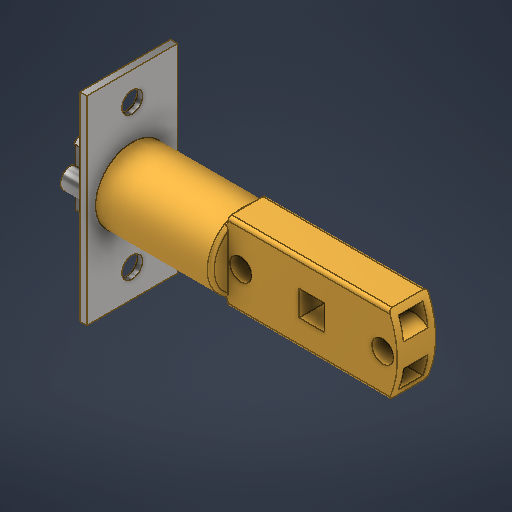
# Autodesk Inventor part: LOK-58 LLAVIN DE POMO (PASADOR)
Saved by Autodesk Inventor 2025 (Build 290162000, 162)
## iProperties
Created: 2026-02-18
Part Number: LOK-58 LLAVIN DE POMO (PASADOR)
Material: Latón, amarillo claro
Document SubType Name: Modeling
Designer: ROLANDO
Density: 8.47 g/cm^3
Appearance: Latón - Satinado
Author: ROLANDO
Autodesk Inventor part; units mm, degrees
ref_plane "YZ Plane" through (0, 0, 0) normal (1, 0, 0) x (0, 1, 0)
ref_plane "XZ Plane" through (0, 0, 0) normal (0, 1, 0) x (-1, 0, 0)
ref_plane "XY Plane" through (0, 0, 0) normal (0, 0, 1) x (1, 0, 0)
sketch "Boceto1" plane through (0, 0, 0) normal (0, 0, 1) x (1, 0, 0)
  circle A0 centre (20.35, 0) radius 3.15
  circle A1 centre (-20.35, 0) radius 3.15
  line L0 (-3.65, 3.65) -> (3.65, 3.65)
  line L1 (3.65, 3.65) -> (3.65, -3.65)
  line L2 (3.65, -3.65) -> (-3.65, -3.65)
  line L3 (-3.65, -3.65) -> (-3.65, 3.65)
  line L4 (-3.65, 3.65) -> (3.65, -3.65) construction
  line L5 (3.65, 3.65) -> (-3.65, -3.65) construction
  line L6 (-24, 11.25) -> (22, 11.25)
  line L7 (22, -11.25) -> (-24, -11.25)
  line L8 (-24, -11.25) -> (-24, 11.25)
  arc A2 (22, -11.25) -> (22, 11.25) centre (-2.0625, 0) ccw
  point P0 (0, 0)
  point P1 (0, 0)
  point P2 (0, 0)
  dimension "d1" = 6.3
  dimension "d2" = 6.3
  dimension "d3" = 7.3
  dimension "d4" = 7.3
  dimension "d7" = 46
  dimension "d8" = 24
  dimension "d9" = 22.5
  dimension "d10" = 11.25
  dimension "d12" = 1
  dimension "d13" = 46
  dimension "d15" = 3.65
  dimension "d16" = 40.7
  dimension "d17" = 20.35
  constraints: 18 end point, 3 centre point, 2 coincident, 2 horizontal, 2 horizontal alignment, 2 midpoint, 2 parallel, 2 perpendicular, 2 point on circle
  measures "d1" diameter of A0
  measures "d2" diameter of A1
  measures "d3" distance of L1.end L2.end
  measures "d4" distance of L0.end L1.end
  measures "d7" distance of L7.start L7.end
  measures "d8" distance from line of point (0, 0) L8
  measures "d9" distance of L7.end L6.start
  measures "d10" distance from line of point (0, 0) L6
  measures "d13" distance of L6.start L6.end
  measures "d15" distance from line of A1.centre L8
  measures "d16" distance of A1.centre A0.centre
  measures "d17" distance of point (0, 0) A0.centre
extrude "Extrusión1" add sketch "Boceto1" against normal blind 11
sketch "Boceto2" plane through (-24, -11.25, 0) normal (-1, 0, 0) x (0, 0, 1)
  circle A0 centre (-5.5, 11.25) radius 10.5
  line L0 (0, 0) -> (-11, 0) projected
  line L1 (0, 22.5) -> (0, 0) projected
  point P0 (0, 11.25)
  dimension "d20" = 21
  dimension "d21" = 11.25
  dimension "d22" = 5.5
  constraints: 1 centre point
  measures "d20" diameter of A0
  measures "d21" distance from line of L0 A0.centre
  measures "d22" distance from line of L1 A0.centre
extrude "Extrusión2" add sketch "Boceto2" along normal blind 33
sketch "Boceto3" plane through (-57, 0, -5.5) normal (-1, 0, 0) x (0, 0, 1)
  line L0 (-13, 28.5) -> (13, 28.5)
  line L1 (13, 28.5) -> (13, -28.5)
  line L2 (13, -28.5) -> (-13, -28.5)
  line L3 (-13, -28.5) -> (-13, 28.5)
  line L4 (-13, 28.5) -> (13, -28.5) construction
  line L5 (13, 28.5) -> (-13, -28.5) construction
  circle A0 centre (0, 0) radius 10.5 projected
  line L6 (6.5, -8.2462) -> (6.5, -3.1943)
  line L7 (6.5, 8.2462) -> (6.5, 3.1943)
  line L8 (10.2924, 0) -> (-1.6343, 0) construction
  arc A1 (6.5, -3.1943) -> (6.5, 3.1943) centre (7, 0) ccw
  arc A2 (6.5, -8.2462) -> (6.5, 8.2462) centre (0, 0) ccw construction
  point P0 (5.5, 0)
  dimension "d25" = 26
  dimension "d26" = 57
  dimension "d27" = 13
  dimension "d29" = 28.5
  dimension "d68" = 6.5
  dimension "d69" = 3.2332
  dimension "d72" = 0.5
  constraints: 18 end point, 4 point on circle, 2 centre point, 2 horizontal, 2 midpoint, 2 parallel, 1 collinear, 1 perpendicular, 1 point on line, 1 vertical
  measures "d25" distance of L1.end L2.end
  measures "d26" distance of L0.end L1.end
  measures "d27" distance from line of A0.centre L1
  measures "d29" distance from line of L0 A0.centre
  measures "d68" distance from line of point (0, 0) L6
  measures "d69" radius of A1
  measures "d72" distance from line of L6 A1.centre
extrude "Extrusión3" add sketch "Boceto3" along normal blind 2 contours L0 L1 L2 L3 | A0 L6 A1 L7 picked at (7.0604, -6.0073)
shell "Vaciado1" thickness 2 removed faces 1 at (24.4295, -1.9344, -7.3333)
sketch "Boceto4" plane through (-57, 0, -5.5) normal (-1, 0, 0) x (0, 0, 1)
  line L0 (6.5, 2.9943) -> (6.5, -2.9943)
  arc A0 (6.5, -2.9943) -> (6.5, 2.9943) centre (7, 0) ccw
  line L1 (6.3, 8.0853) -> (6.3, -8.0853)
  arc A1 (6.3, 8.0853) -> (6.3, -8.0853) centre (0, 0) ccw
  line L2 (10.2924, 0) -> (-1.6343, 0) construction
  arc A2 (6.5, -8.2462) -> (6.5, 8.2462) centre (0, 0) ccw construction
  point P0 (5.5, 0)
  point P1 (6.5, 0)
  dimension "d41" = 3.0357
  dimension "d42" = 0.5
  dimension "d43" = 0.2
  dimension "d44" = 10.25
  dimension "d45" = 6.3
  constraints: 6 end point, 6 point on circle, 3 centre point, 2 coincident, 2 point on line, 2 vertical, 1 horizontal, 1 midpoint
  measures "d41" radius of A0
  measures "d42" distance from line of L0 A0.centre
  measures "d43" distance between parallel lines of L1 L0
  measures "d44" radius of A1
  measures "d45" distance from line of A1.centre L1
extrude "Extrusión4" add sketch "Boceto4" along normal blind 10.5
fillet "Empalme1" radius 0.5 2 edges at (-67.5, 0, 0.8) (-67.5, 0, 1)
ref_plane "Plano de trabajo4" through (-57, -28.5, -18.5) normal (0, -1, 0) x (1, 0, 0)
sketch "Boceto10" plane through (-57, -28.5, -18.5) normal (0, -1, 0) x (1, 0, 0)
  line L0 (-10.5, 18.8) -> (-10.5, 2.75) projected
  line L1 (0, 19.3) -> (-10, 19.3) projected
  line L2 (0, 2.75) -> (-10.5, 2.75) projected
  line L3 (-2, 0) -> (-2, 26) projected
  line L4 (-10.5, 18.8) -> (-2, 18.8)
  line L5 (-2, 18.8) -> (-2, 2.75)
  arc A0 (-10.5, 18.8) -> (-2, 2.75) centre (7.4843, 18.0486) ccw
  point P0 (57, 18.5)
  point P1 (-10.5, 17.2972)
  dimension "d86" = 18
  constraints: 4 end point, 3 point on line, 2 point on circle, 1 centre point, 1 perpendicular, 1 other
  measures "d86" radius of A0
extrude "Extrusión5" cut sketch "Boceto10" against normal up to surface (57 mm away) contours A0 L2 L0
sketch "Boceto11" plane through (-59, 0, -5.5) normal (-1, 0, 0) x (0, 0, 1)
  circle A0 centre (0, 20.5) radius 3
  line L0 (13, -28.5) -> (13, 28.5) projected
  line L1 (-13, 28.5) -> (-13, -28.5) projected
  line L2 (13, 28.5) -> (-13, 28.5) projected
  circle A1 centre (0, -20.5) radius 3
  line L3 (-13, -28.5) -> (13, -28.5) projected
  point P0 (5.5, 0)
  dimension "d89" = 6
  dimension "d90" = 13
  dimension "d91" = 13
  dimension "d92" = 8
  dimension "d93" = 6
  dimension "d94" = 13
  dimension "d95" = 13
  dimension "d96" = 8
  constraints: 2 centre point
  measures "d89" diameter of A0
  measures "d90" distance from line of L0 A0.centre
  measures "d91" distance from line of L1 A0.centre
  measures "d92" distance from line of L2 A0.centre
  measures "d93" diameter of A1
  measures "d94" distance from line of L0 A1.centre
  measures "d95" distance from line of L1 A1.centre
  measures "d96" distance from line of L3 A1.centre
hole "Agujero1" at (-59, 20.5, -5.5) at (-59, -20.5, -5.5) direction (1, 0, 0) diameter 6 depth 2 tip angle 118 countersink diameter 7 countersink angle 90
fillet "Empalme2" radius 1 9 edges at (-24, 10.5, -5.5) (-24, -5.1235, 3.6652) (-24, 5.1235, 3.6652) (-24, 0, -16) (-24, -10.5, -5.5) (-1, -11.25, 0) (-1, -11.25, -11) (-1, 11.25, -11) (-1, 11.25, 0)
